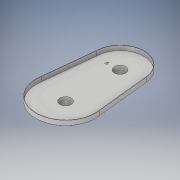
# Autodesk Inventor part: Tampa Capa CVT
Saved by Autodesk Inventor 2019 (Build 230136000, 136)
## iProperties
Created: 2020-05-31
Part Number: Tampa Capa CVT
Material: Genérico
Document SubType Name: Chapa de metal
Designer: andre
Density: 1 g/cm^3
Sheet Metal Rule: Padrão_mm
Appearance: Padrão
Author: andre
Autodesk Inventor part; units mm, degrees
ref_plane "YZ Plane" through (0, 0, 0) normal (1, 0, 0) x (0, 1, 0)
ref_plane "XZ Plane" through (0, 0, 0) normal (0, 1, 0) x (-1, 0, 0)
ref_plane "XY Plane" through (0, 0, 0) normal (0, 0, 1) x (1, 0, 0)
sketch "Esboço1" plane through (0, 0, 0) normal (0, 1, 0) x (-1, 0, 0)
  arc A0 (128.4825, -19.8053) -> (-128.4825, -19.8053) centre (0, 0) ccw
  arc A1 (130, -19.8053) -> (-130, -19.8053) centre (0, 0) ccw
  line L0 (0, 0) -> (0, -241) construction
  arc A2 (-104.9999, -240.8364) -> (105, -241) centre (0, -241) ccw
  arc A3 (-106.5, -241) -> (106.5, -241) centre (0, -241) ccw
  line L1 (130, -19.8053) -> (106.5, -241)
  line L2 (-130, -19.8053) -> (-106.5, -241)
  line L3 (128.4825, -19.8053) -> (105, -241)
  line L4 (-128.4825, -19.8053) -> (-104.9999, -240.8364)
  dimension "d0" = 260
  dimension "d1" = 263
  dimension "d2" = 241
  dimension "d3" = 210
  dimension "d4" = 213
  constraints: 10 end point, 8 point on circle, 4 centre point, 4 coincident, 1 parallel, 1 vertical
  measures "d0" diameter of A0
  measures "d1" diameter of A1
  measures "d2" distance of L0.start L0.end
  measures "d3" diameter of A2
  measures "d4" diameter of A3
extrude "Extrusão1" add sketch "Esboço1" along normal blind 1.5 contours L3 A2 L4 A0
sketch "Esboço2" plane through (0, 1.5, 0) normal (0, 1, 0) x (1, 0, 0)
  arc A0 (-130, 19.8053) -> (129.9878, 19.8852) centre (0, 0) ccw
  line L0 (0, 0) -> (0, 241) construction
  arc A1 (105.9327, 251.9775) -> (-105.9324, 251.9811) centre (0, 241) ccw
  line L1 (-130, 19.8053) -> (-105.9324, 251.9811)
  arc A2 (-128.4825, 19.8053) -> (128.4825, 19.8053) centre (0, 0) ccw projected
  line L2 (-128.4825, 19.8053) -> (-105, 241)
  arc A3 (104.9999, 240.8364) -> (-105, 241) centre (0, 241) ccw projected
  line L3 (105.9324, 251.9811) -> (129.9878, 19.8852)
  line L4 (128.4825, 19.8053) -> (104.9999, 240.8364) projected
  line L5 (128.4825, 19.8053) -> (104.9999, 240.8364)
  dimension "d7" = 263
  dimension "d8" = 241
  dimension "d9" = 213
  constraints: 10 end point, 6 point on circle, 2 centre point, 2 coincident, 1 collinear, 1 point on line, 1 tangent, 1 vertical
  measures "d7" diameter of A0
  measures "d8" distance of L0.start L0.end
  measures "d9" diameter of A1
extrude "Extrusão2" add sketch "Esboço2" along normal blind 20
sketch "Esboço3" plane through (0, 1.5, 0) normal (0, 1, 0) x (1, 0, 0)
  circle A0 centre (0, 0) radius 25
  line L0 (0, 0) -> (0, 241)
  circle A1 centre (0, 241) radius 25
  dimension "d12" = 50
  dimension "d13" = 241
  dimension "d14" = 50
  constraints: 2 centre point, 2 coincident, 2 end point, 1 vertical
  measures "d12" diameter of A0
  measures "d13" distance of L0.start L0.end
  measures "d14" diameter of A1
extrude "Extrusão3" cut sketch "Esboço3" against normal blind 20
sketch "Esboço4" plane through (0, 0, 0) normal (0, -1, 0) x (1, 0, 0)
  circle A0 centre (0, 0) radius 26.5
  line L0 (0, 0) -> (0, -241)
  circle A1 centre (0, -241) radius 26.5
  circle A2 centre (0, 0) radius 25
  circle A3 centre (0, -241) radius 25
  dimension "d17" = 53
  dimension "d18" = 241
  dimension "d19" = 53
  dimension "d20" = 50
  dimension "d21" = 50
  constraints: 4 centre point, 4 coincident, 2 end point, 1 vertical
  measures "d17" diameter of A0
  measures "d18" distance of L0.start L0.end
  measures "d19" diameter of A1
  measures "d20" diameter of A2
  measures "d21" diameter of A3
extrude "Extrusão4" add sketch "Esboço4" along normal blind 40
sketch "Esboço5" plane through (0, 1.5, 0) normal (0, 1, 0) x (1, 0, 0)
  point P0 (0, 0)
sketch "Esboço6" plane through (0, 0, 0) normal (0, -1, 0) x (1, 0, 0)
  point P0 (0, 0)
sketch "Esboço7" plane through (0, 0, 0) normal (0, -1, 0) x (1, 0, 0)
  circle A0 centre (0, -241) radius 25 projected
  circle A1 centre (-55, -241) radius 3.5
  point P0 (0, 0)
  dimension "d24" = 7
  dimension "d25" = 55
  constraints: 1 centre point, 1 coincident
  measures "d24" diameter of A1
  measures "d25" distance of point (0, -241) A1.centre
extrude "Extrusão5" cut sketch "Esboço7" against normal blind 10 contours A1
sketch "Esboço8" plane through (0, 0, 0) normal (0, -1, 0) x (1, 0, 0)
  circle A0 centre (-51, -233.5) radius 1.65
  circle A1 centre (-59, -233.5) radius 1.65
  circle A2 centre (-55, -241) radius 3.5 projected
  circle A3 centre (-55, -241) radius 3.5
  point P0 (0, 0)
  dimension "d28" = 3.3
  dimension "d29" = 3.3
  dimension "d50" = 7.5
  dimension "d51" = 4
  dimension "d52" = 7.5
  dimension "d53" = 4
  constraints: 3 centre point, 1 coincident
  measures "d28" diameter of A0
  measures "d29" diameter of A1
  measures "d50" vertical distance of A1.centre A3.centre
  measures "d51" horizontal distance of A3.centre A1.centre
  measures "d52" vertical distance of A3.centre A0.centre
  measures "d53" horizontal distance of A3.centre A0.centre
extrude "Extrusão6" cut sketch "Esboço8" against normal blind 10 contours A0 | A1
equation "\"Raio_vergadura\" = Espessura"
equation "\"Largura_alívio_de_vergadura\" = Espessura"
equation "\"Profundidade_alívio_de_vergadura\" = 0.5 * Espessura"
equation "\"Tamanho_alívio_de_dobra\" = 4 * Espessura"
equation "\"Remanescente_mínimo\" = 2 * Espessura"
equation "\"Raiodetransição\" = Raio_vergadura"
equation "\"Tamanho_de_raio_de_Jacobi\" = Raio_vergadura"
equation "\"TamanhoFolga\" = Espessura"
equation "\"Espessura\" = 0.5"
